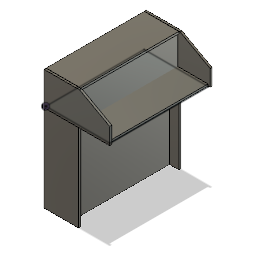
2 manuals_v4 (Autodesk Fusion 360 design; units mm, degrees)
Autodesk Fusion 360 part; units mm, degrees
sketch "Sketch1" plane through (0, 0, 0) normal (0, 1, 0) x (1, 0, 0)
  line L0 (0, -20) -> (-182, -20)
  line L1 (-182, -20) -> (-182, 827)
  line L2 (-182, 827) -> (0, 827)
  line L3 (0, 827) -> (0, -20)
  dimension "d1" = 182
  dimension "d2" = 847
  constraint horizontal L0
  constraint vertical L1
  constraint horizontal L2
  constraint vertical L3
  measures "d1" distance of L0.start L0.end
  measures "d2" distance of L0.start L2.end
extrude "Extrude1" add sketch "Sketch1" along normal blind 18 makes body 1
sketch "Sketch2" plane through (0, 0, 0) normal (0, 0, 1) x (1, 0, 0)
  line L0 (-182, 0, 20) -> (118, 0, 20)
  line L1 (118, 0, 20) -> (118, 750, 20)
  line L2 (118, 750, 20) -> (-182, 750, 20)
  line L3 (-182, 750, 20) -> (-182, 0, 20)
  point P0 (-182, 0)
  dimension "d5" = 300
  dimension "d6" = 750
extrude "Extrude2" add sketch "Sketch2" along normal blind 18 separate body contours L0 L1 L2 L3 in plane through (0, 0, 20) normal (0, 0, 1) makes body 2
copy_body "CopyPasteBodies1" bodies 2 makes body 3
move_body "Move1" bodies 3 to x (1, 0, 0) y (0, 1, 0) z (0, 0, 1) at (0, 0, -865)
sketch "Sketch3" plane through (0, 0, 0) normal (1, 0, 0) x (0, 0, -1)
  line L0 (-20, 0) -> (827, 0)
  line L1 (827, 0) -> (827, 750)
  line L2 (827, 750) -> (-20, 750)
  line L3 (-20, 750) -> (-20, 0)
  point P0 (-20, 0)
  dimension "d9" = 847
  dimension "d10" = 750
  constraint horizontal L0
  constraint vertical L1
  constraint horizontal L2
  constraint vertical L3
  constraint coincident P0 L0.start
  measures "d9" distance of P0 L0.end
  measures "d10" distance of P0 L2.end
extrude "Extrude3" add sketch "Sketch3" along normal blind 18 separate body makes body 4
move_body "Move2" bodies 2 3 to x (1, 0, 0) y (0, 1, 0) z (0, 0, 1) at (-18, 0, 0)
copy_body "CopyPasteBodies2" bodies 4 makes body 5
move_body "Move3" bodies 5 to x (1, 0, 0) y (0, 1, 0) z (0, 0, 1) at (-200, 0, 0)
sketch "Sketch4" plane through (0, 0, 0) normal (0, 1, 0) x (1, 0, 0)
  line L0 (-200, -20, 750) -> (350, -20, 750)
  line L1 (350, -20, 750) -> (350, 827, 750)
  line L2 (350, 827, 750) -> (-200, 827, 750)
  line L3 (-200, 827, 750) -> (-200, -20, 750)
  point P0 (-200, -20)
  dimension "d13" = 550
  dimension "d14" = 847
extrude "Extrude5" add sketch "Sketch4" along normal blind 18 separate body contours L0 L1 L2 L3 in plane through (0, 750, 0) normal (0, 1, 0) makes body 6
sketch "Sketch6" plane through (0, 0, 0) normal (0, 0, 1) x (1, 0, 0)
  line L0 (-200, 750, -845) -> (368, 750, -845)
  line L1 (368, 750, -845) -> (368, 1036, -845)
  line L2 (368, 1036, -845) -> (-200, 1036, -845)
  line L3 (-200, 1036, -845) -> (-200, 750, -845)
  line L4 (368, 893, -845) -> (109.2529, 1036, -845)
  point P0 (-200, 750)
  dimension "d21" = 568
  dimension "d22" = 286
extrude "Extrude6" add sketch "Sketch6" along normal blind 18 separate body contours L0 L1 L2 L3 L4 in plane through (0, 0, -845) normal (0, 0, 1) makes body 7
copy_body "CopyPasteBodies3" bodies 7 makes body 8
move_body "Move4" bodies 8 to x (1, 0, 0) y (0, 1, 0) z (0, 0, 1) at (0, 0, 865)
sketch "Sketch7" plane through (0, 0, 0) normal (1, 0, 0) x (0, 0, -1)
  line L0 (827, 768, -200) -> (-20, 768, -200)
  line L1 (-20, 768, -200) -> (-20, 1027.4058, -200)
  line L2 (-20.0261, 1018, -200) -> (827, 1018, -200)
  line L3 (827, 1018, -200) -> (827, 768, -200)
  point P0 (827, 768)
  dimension "d25" = 847
  dimension "d26" = 250
extrude "Extrude7" add sketch "Sketch7" along normal blind 18 separate body contours L0 L1 L2 L3 in plane through (-200, 0, 0) normal (1, 0, 0) makes body 9
sketch "Sketch8" plane through (0, 0, 0) normal (0, 1, 0) x (1, 0, 0)
  line L0 (-182, -20, 1018) -> (118, -20, 1018)
  line L1 (118, -20, 1018) -> (118, 827, 1018)
  line L2 (118, 827, 1018) -> (-182, 827, 1018)
  line L3 (-182, 827, 1018) -> (-182, -20, 1018)
  point P0 (-182, -20)
  dimension "d29" = 300
  dimension "d30" = 847
extrude "Extrude8" add sketch "Sketch8" against normal blind 18 separate body contours L0 L1 L2 L3 in plane through (0, 1018, 0) normal (0, 1, 0) makes body 10
sketch "Sketch9" plane through (0, 0, 0) normal (1, 0, 0) x (0, 0, -1)
  line L0 (-20, 1018, 118) -> (827, 1018, 118)
  line L1 (827, 1018, 118) -> (827, 768, 118)
  line L2 (827, 768, 118) -> (-20, 768, 118)
  line L3 (-20, 768, 118) -> (-20, 1018, 118)
  point P0 (-20, 1018)
  dimension "d33" = 847
  dimension "d34" = 250
extrude "Extrude9" add sketch "Sketch9" along normal blind 18 separate body contours L0 L1 L2 L3 in plane through (118, 0, 0) normal (1, 0, 0) makes body 11
sketch "Sketch10" plane through (0, 0, 20) normal (0, 0, -1) x (-1, 0, 0)
  line L0 (200, 750) -> (200, 1036)
  line L1 (200, 1036) -> (-109.2529, 1036)
  line L2 (-368, 893) -> (-368, 750)
  line L3 (-368, 750) -> (200, 750)
  line L4 (-118, 1018) -> (-188.7107, 947.2893)
  line L5 (-118, 1018) -> (-18, 1018) construction
  line L6 (-188.7107, 947.2893) -> (-166.7107, 947.2893)
  line L7 (-166.7107, 947.2893) -> (-118, 1000)
  line L8 (-118, 1000) -> (-118, 1018)
  line L9 (-109.2529, 1036) -> (-368, 893)
  point P0 (-118, 1018)
  point P1 (-118, 1000)
  dimension "d37" = 135
  dimension "d38" = 100
  dimension "d39" = 22
  constraint horizontal L5
  constraint coincident P0 L4.start
  constraint parallel L1 L6
  constraint coincident P1 L7.end
  measures "d37" angle of L4 L5
  measures "d38" distance of P0 L4.end
  measures "d39" distance of L4.end L6.end
extrude "Extrude10" add sketch "Sketch10" along normal blind 847 separate body contours L4 L6 L7 L8 makes body 12
move_body "Move5" bodies 10 to x (1, 0, 0) y (0, 1, 0) z (0, 0, 1) at (-29.4627, 12.1302, 1.6956)
move_body "Move6" bodies 10 to x (1, 0, 0) y (0, 1, 0) z (0, 0, 1) at (0, -6.3189, 0)
move_body "Move7" bodies 11 to x (1, 0, 0) y (0, 1, 0) z (0, 0, 1) at (-48.5711, -10.2873, -2.0674)
move_body "Move8" bodies 10 to x (1, 0, 0) y (0, 1, 0) z (0, 0, 1) at (12.2277, 4.2236, -0.12)
move_body "Move9" bodies 10 to x (1, 0, 0) y (0, 1, 0) z (0, 0, 1) at (0, -2.0384, 0)
move_body "Move10" bodies 9 to x (1, 0, 0) y (0, 1, 0) z (0, 0, 1) at (0, -3.28, 0)
move_body "Move11" bodies 10 to x (1, 0, 0) y (0, 1, 0) z (0, 0, 1) at (0, 10.6207, 0)
hidden bodies 12
